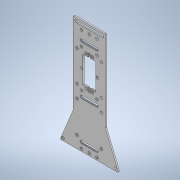
# Autodesk Inventor part: Рама
Saved by Autodesk Inventor 2021 (Build 250183000, 183)
## iProperties
Created: 2022-07-08
Part Number: Рама
Material: Типовые
Document SubType Name: Modeling
Designer: zvi20
Density: 1 g/cm^3
Appearance: По умолчанию
Author: zvi20
Autodesk Inventor part; units mm, degrees
ref_plane "YZ Plane" through (0, 0, 0) normal (1, 0, 0) x (0, 1, 0)
ref_plane "XZ Plane" through (0, 0, 0) normal (0, 1, 0) x (-1, 0, 0)
ref_plane "XY Plane" through (0, 0, 0) normal (0, 0, 1) x (1, 0, 0)
sketch "Эскиз1" plane through (0, 0, 0) normal (0, 0, 1) x (1, 0, 0)
  line L0 (13.2469, -7.2038) -> (61.2469, -7.2038)
  line L1 (62.2469, -8.2038) -> (62.2469, -134.2038)
  line L2 (81.2561, -184.2038) -> (-6.7623, -184.2038)
  line L3 (12.2469, -134.2038) -> (12.2469, -8.2038)
  line L4 (-7.6876, -182.8244) -> (12.2469, -134.2038)
  line L5 (62.2469, -134.2038) -> (82.1813, -182.8244)
  circle A0 centre (25.2469, -180.2038) radius 2
  circle A1 centre (78.2469, -180.2038) radius 2
  arc A2 (-7.6876, -182.8244) -> (-6.7623, -184.2038) centre (-6.7623, -183.2038) ccw
  arc A3 (81.2561, -184.2038) -> (82.1813, -182.8244) centre (81.2561, -183.2038) ccw
  arc A4 (62.2469, -8.2038) -> (61.2469, -7.2038) centre (61.2469, -8.2038) ccw
  arc A5 (13.2469, -7.2038) -> (12.2469, -8.2038) centre (13.2469, -8.2038) ccw
  arc A6 (57.7469, -14.2038) -> (57.7469, -10.2038) centre (57.7469, -12.2038) ccw
  arc A7 (16.7469, -10.2038) -> (16.7469, -14.2038) centre (16.7469, -12.2038) ccw
  line L6 (16.7469, -10.2038) -> (57.7469, -10.2038)
  line L7 (57.7469, -14.2038) -> (16.7469, -14.2038)
  circle A8 centre (49.2469, -20.2038) radius 2
  line L8 (38.7469, -45.7038) -> (35.7469, -45.7038)
  line L9 (38.7469, -45.7038) -> (38.7469, -51.7038)
  line L10 (38.7469, -51.7038) -> (47.2469, -51.7038)
  line L11 (47.2469, -51.7038) -> (47.2469, -92.7038)
  line L12 (47.2469, -92.7038) -> (38.7469, -92.7038)
  line L13 (38.7469, -92.7038) -> (38.7469, -98.7038)
  line L14 (38.7469, -98.7038) -> (35.7469, -98.7038)
  line L15 (35.7469, -98.7038) -> (35.7469, -92.7038)
  line L16 (35.7469, -92.7038) -> (27.2469, -92.7038)
  line L17 (27.2469, -92.7038) -> (27.2469, -51.7038)
  line L18 (27.2469, -51.7038) -> (35.7469, -51.7038)
  line L19 (35.7469, -51.7038) -> (35.7469, -45.7038)
  circle A9 centre (24.7469, -72.2038) radius 2
  circle A10 centre (49.7469, -72.2038) radius 2
  arc A11 (25.2469, -32.2038) -> (25.2469, -36.2038) centre (25.2469, -34.2038) ccw
  line L20 (25.2469, -32.2038) -> (49.2469, -32.2038)
  line L21 (25.2469, -36.2038) -> (49.2469, -36.2038)
  arc A12 (49.2469, -36.2038) -> (49.2469, -32.2038) centre (49.2469, -34.2038) ccw
  arc A13 (49.2469, -36.2038) -> (49.2469, -32.2038) centre (49.2469, -34.2038) ccw
  circle A14 centre (42.2469, -48.2038) radius 2
  circle A15 centre (49.2469, -42.7038) radius 2
  circle A16 centre (56.2469, -48.2038) radius 2
  circle A17 centre (32.2469, -48.2038) radius 2
  circle A18 centre (25.2469, -42.7038) radius 2
  circle A19 centre (18.2469, -48.2038) radius 2
  arc A20 (25.2469, -108.2038) -> (25.2469, -112.2038) centre (25.2469, -110.2038) ccw
  line L22 (25.2469, -112.2038) -> (49.2469, -112.2038)
  line L23 (25.2469, -108.2038) -> (49.2469, -108.2038)
  arc A21 (49.2469, -112.2038) -> (49.2469, -108.2038) centre (49.2469, -110.2038) ccw
  arc A22 (49.2469, -112.2038) -> (49.2469, -108.2038) centre (49.2469, -110.2038) ccw
  circle A23 centre (42.2469, -96.2038) radius 2
  circle A24 centre (49.2469, -101.7038) radius 2
  circle A25 centre (56.2469, -96.2038) radius 2
  circle A26 centre (18.2469, -96.2038) radius 2
  circle A27 centre (32.2469, -96.2038) radius 2
  circle A28 centre (25.2469, -101.7038) radius 2
  circle A29 centre (56.2469, -116.2038) radius 2
  circle A30 centre (18.2469, -116.2038) radius 2
  arc A31 (49.2469, -173.2038) -> (49.2469, -169.2038) centre (49.2469, -171.2038) ccw
  arc A32 (25.2469, -169.2038) -> (25.2469, -173.2038) centre (25.2469, -171.2038) ccw
  line L24 (25.2469, -169.2038) -> (49.2469, -169.2038)
  line L25 (25.2469, -173.2038) -> (49.2469, -173.2038)
  circle A33 centre (49.2469, -180.2038) radius 2
  circle A34 centre (37.2469, -180.2038) radius 2
  circle A35 centre (56.2469, -165.2038) radius 2
  circle A36 centre (18.2469, -165.2038) radius 2
  circle A37 centre (-3.7531, -180.2038) radius 2
  circle A38 centre (37.2469, -20.2038) radius 2
  circle A39 centre (25.2469, -20.2038) radius 2
  point P0 (0, 0)
  point P1 (82.7469, -184.2038)
  point P2 (-8.2531, -184.2038)
  constraints: 52 end point, 40 centre point, 28 point on circle, 11 tangent, 10 point on line, 5 perpendicular, 4 horizontal, 3 equal radius, 1 vertical
extrude "Выдавливание2" add sketch "Эскиз1" along normal blind 2
